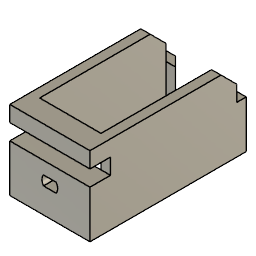
servo_holder (Autodesk Fusion 360 design; units mm, degrees)
part number: 2025-10-28-16-11-16-765
Autodesk Fusion 360 part; units mm, degrees
sketch "Schizzo1" plane through (0, 0, 0) normal (0, 0, 1) x (1, 0, 0)
  line L0 (12.7, -24.75) -> (-12.7, -24.75)
  line L1 (-12.7, -24.75) -> (-12.7, 24.75)
  line L2 (12.7, 24.75) -> (12.7, -24.75)
  line L3 (12.7, -24.75) -> (-12.7, 24.75) construction
  line L4 (-12.7, -24.75) -> (12.7, 24.75) construction
  line L5 (9.7, -18.25) -> (-9.7, -18.25)
  line L6 (9.7, 21.75) -> (9.7, -18.25)
  line L7 (-9.7, -18.25) -> (-9.7, 21.75)
  line L8 (-12.7, 24.75) -> (-9.7, 24.75)
  line L9 (9.7, 24.75) -> (12.7, 24.75)
  line L10 (-9.7, 21.75) -> (-6.7, 21.75)
  line L11 (-6.7, 21.75) -> (-9.7, 24.75)
  line L12 (9.7, 21.75) -> (6.7, 21.75)
  line L13 (6.7, 21.75) -> (9.7, 24.75)
  line L14 (-9.7, -18.25) -> (-12.7, -18.25)
  line L15 (9.7, -18.25) -> (12.7, -18.25)
  line L16 (-9.7, 21.75) -> (-12.7, 21.75)
  line L17 (9.7, 21.75) -> (12.7, 21.75)
  dimension "d15" = 19.4
  dimension "d16" = 3
  dimension "d17" = 3
  dimension "d18" = 6.5
  dimension "d19" = 43
  dimension "d20" = 3
  dimension "d22" = 3
  dimension "d23" = 3
  dimension "d24" = 3
  constraint horizontal L0
  constraint perpendicular L0 L1
  constraint parallel L0 L8
  constraint parallel L1 L2
  constraint coincident L3 origin
  constraint coincident L4 origin
  constraint perpendicular L7 L8
  constraint coincident L9.start L8
  constraint collinear L8 L9
  constraint coincident L5 L7.start
  constraint perpendicular L7 L10
  constraint perpendicular L6 L12
  constraint vertical L8.end L7.end
  constraint vertical L9.start L6.start
  constraint coincident L1 L14.end
  constraint perpendicular L1 L14
  constraint coincident L2 L15.end
  constraint perpendicular L2 L15
  constraint coincident L1 L16.end
  constraint perpendicular L1 L16
  constraint coincident L2 L17.end
  constraint perpendicular L2 L17
  measures "d15" distance of L5.start L5.end
  measures "d16" distance of L1 L7
  measures "d17" distance of L2 L6
  measures "d18" distance of L0 L5
  measures "d19" distance of L5.start L9.start
  measures "d20" distance of L7.end L10.end
  measures "d22" distance of L6.start L12.end
  measures "d23" distance of L8 L10
  measures "d24" distance of L9 L12
extrude "Estrusione2" add sketch "Schizzo1" along normal blind 25 contours L0 L1 L2 L5 L14 L15 | L2 L6 L15 L17 | L1 L7 L14 L16
extrude "Estrusione3" add sketch "Schizzo1" along normal blind 15 contours L2 L9 L12 L13 L17 | L1 L8 L10 L11 L16
extrude "Estrusione4" cut sketch "Schizzo1" along normal blind 5 from surface at 15 contours L0 L1 L2 L5 L14 L15
chamfer "Smusso1" distance 5 angle 45 2 edges at (11.2, 21.75, 25) (-11.2, 21.75, 25)
sketch "Schizzo2" plane through (0, -24.75, 0) normal (0, -1, 0) x (1, 0, 0)
  line L0 (12.7, 15) -> (-12.7, 15)
  line L1 (-12.7, 15) -> (-12.7, 0)
  line L2 (-12.7, 0) -> (12.7, 0)
  line L3 (12.7, 0) -> (12.7, 15)
  line L4 (0, 15) -> (0, 0) construction
  circle A0 centre (0, 9.5) radius 2.5
  line L5 (-2, 11) -> (2, 11)
  line L6 (-2, 8) -> (2, 8)
  line L7 (-2.5, 9.5) -> (2.5, 9.5) construction
  dimension "d33" = 5
  dimension "d34" = 3
  dimension "d35" = 3
  constraint midpoint L0 L4.start
  constraint coincident L4.end origin
  constraint coincident L4 A0.centre
  constraint coincident A0 L5.start
  constraint perpendicular L4 L5
  constraint coincident A0 L6.start
  constraint coincident A0 L6.end
  constraint perpendicular L4 L6
  constraint coincident A0 L5.end
  constraint coincident A0 L7.end
  constraint perpendicular L4 L7
  constraint coincident A0 L7.start
  constraint coincident A0.centre L7
  constraint symmetric L5 L6 L7
  measures "d33" diameter of A0
  measures "d34" distance of L4.start A0
  measures "d35" distance of L5 L6
extrude "Estrusione5" cut sketch "Schizzo2" against normal blind 5 contours A0 L5 L6
equation "d17 = d16"
equation "d20 = spessore"
equation "spessore = 3 mm"
equation "d22 = spessore"
equation "d23 = spessore"
equation "d24 = spessore"
